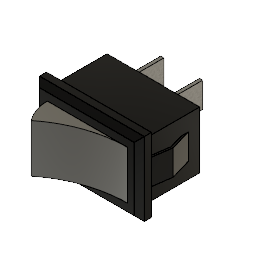
Irrigation unit - Rectangular On-off switch v1 (Autodesk Fusion 360 design; units mm, degrees)
Autodesk Fusion 360 part; units mm, degrees
note: some values were not read from the file. Set by a fixed rule: which face or edge a step refers to.
sketch "Sketch1" plane through (0, 0, 0) normal (0, 1, 0) x (1, 0, 0)
  line L0 (-0.7248, -15.1125) -> (17.4752, -15.1125)
  line L1 (17.4752, -15.1125) -> (17.4752, -3.8625)
  line L2 (17.4752, -3.8625) -> (-0.7248, -3.8625)
  line L3 (-0.7248, -3.8625) -> (-0.7248, -15.1125)
  line L4 (-1.9398, -16.7375) -> (18.6902, -16.7375)
  line L5 (18.6902, -16.7375) -> (18.6902, -2.2375)
  line L6 (18.6902, -2.2375) -> (-1.9398, -2.2375)
  line L7 (-1.9398, -2.2375) -> (-1.9398, -16.7375)
  line L8 (18.6902, -9.4875) -> (-20.1398, -9.4875) construction
  line L9 (8.3752, -16.7375) -> (8.3752, -13.4875) construction
  dimension "d727" = 18.2
  dimension "d728" = 11.25
  dimension "d729" = 14.5
  dimension "d730" = 20.63
  measures "d727" distance of L1 L3
  measures "d728" distance of L0 L2
  measures "d729" distance of L4 L6
  measures "d730" distance of L5 L7
extrude "Extrude1" add sketch "Sketch1" along normal blind 10.7 contours L0 L1 L2 L3 makes body 1
extrude "Extrude2" add sketch "Sketch1" against normal blind 2.4 contours L0 L1 L2 L3 | L4 L5 L6 L7 bodies 1
chamfer "Chamfer1" distance 1 angle 45 4 edges at (8.3752, -2.4, 16.7375) (-1.9398, -2.4, 9.4875) (8.3752, -2.4, 2.2375) (18.6902, -2.4, 9.4875) on bodies 1
sketch "Sketch2" plane through (17.4752, 0, 0) normal (1, 0, 0) x (0, 0, -1)
  line L0 (-15.1125, 0) -> (-3.8625, 0)
  line L1 (-3.8625, 0) -> (-3.8625, 10.7)
  line L2 (-3.8625, 10.7) -> (-15.1125, 10.7)
  line L3 (-15.1125, 10.7) -> (-15.1125, 0)
  line L4 (-11.9875, 0) -> (-6.9875, 0)
  line L5 (-6.9875, 0) -> (-6.9875, 8.5)
  line L6 (-6.9875, 8.5) -> (-11.9875, 8.5)
  line L7 (-11.9875, 8.5) -> (-11.9875, 0)
  line L8 (-16.7375, 0) -> (-2.2375, 0)
  dimension "d736" = 8.5
  dimension "d737" = 5
  measures "d736" distance of L6 L8
  measures "d737" distance of L5 L7
extrude "Extrude3" add sketch "Sketch2" along normal up to surface (1.215 mm away) separate body contours L0 L4 L5 L6 L7 L8 makes body 2
sketch "Sketch3" plane through (0, 0, 11.9875) normal (0, 0, 1) x (1, 0, 0)
  line L0 (18.6902, 0) -> (18.6902, 8.5)
  line L1 (18.6902, 8.5) -> (17.4752, 8.5)
  line L2 (18.6902, 4.25) -> (17.4752, 8.5)
  line L3 (18.6902, 4.25) -> (18.0827, 0)
  line L4 (17.4752, 7.0861) -> (18.2811, 4.2671)
  line L5 (18.2811, 4.2671) -> (17.5547, -0.8149)
  line L6 (17.4752, 8.5) -> (17.4752, 0)
  line L7 (17.4752, 0) -> (18.6902, 0)
extrude "Extrude5" cut sketch "Sketch3" against normal up to surface (5 mm away) contours L0 L3 L7 | L0 L1 L2 | L4 L5 L6 L7 bodies 2
copy_body "CopyPasteBodies1" bodies 2 makes body 3
move_body "Move1" bodies 3 to x (-1, 0, 0) y (0, 1, 0) z (0, 0, -1) at (34.9503, 0, 13.9751)
move_body "Move2" bodies 3 to x (1, 0, 0) y (0, 1, 0) z (0, 0, 1) at (-18.004, 0, 5)
combine "Combine1" operation add target body 1 tool bodies 2 3
sketch "Sketch4" plane through (0, 10.7, 0) normal (0, 1, 0) x (-1, 0, 0)
  line L0 (0.7248, 3.8625) -> (0.7248, 15.1125)
  line L1 (0.7248, 15.1125) -> (-17.4752, 15.1125)
  line L2 (-17.4752, 15.1125) -> (-17.4752, 3.8625)
  line L3 (-17.4752, 3.8625) -> (0.7248, 3.8625)
  line L4 (-1.8252, 11.9875) -> (-2.4752, 11.9875)
  line L5 (-2.4752, 11.9875) -> (-2.4752, 6.9875)
  line L6 (-2.4752, 6.9875) -> (-1.8252, 6.9875)
  line L7 (-1.8252, 6.9875) -> (-1.8252, 11.9875)
  line L8 (0.7248, 3.8625) -> (0.7248, 15.1125)
  line L9 (-18.6902, 9.4875) -> (20.1398, 9.4875)
  dimension "d744" = 0.65
  dimension "d745" = 5
  dimension "d746" = 3.2
  measures "d744" distance of L5 L7
  measures "d745" distance of L4 L6
  measures "d746" distance of L5 L8
extrude "Extrude6" add sketch "Sketch4" along normal blind 8 separate body contours L4 L5 L7 L9 | L5 L6 L7 L9 makes body 4
copy_body "CopyPasteBodies2" bodies 4 makes body 5
move_body "Move3" bodies 5 to x (1, 0, 0) y (0, 1, 0) z (0, 0, 1) at (7.6, 0, 0)
sketch "Sketch5" plane through (0, -2.4, 0) normal (0, -1, 0) x (1, 0, 0)
  line L0 (-0.9398, 3.2375) -> (17.6902, 3.2375)
  line L1 (17.6902, 3.2375) -> (17.6902, 15.7375)
  line L2 (17.6902, 15.7375) -> (-0.9398, 15.7375)
  line L3 (-0.9398, 15.7375) -> (-0.9398, 3.2375)
  line L4 (0.3752, 4.7375) -> (16.3752, 4.7375)
  line L5 (16.3752, 4.7375) -> (16.3752, 14.2375)
  line L6 (16.3752, 14.2375) -> (0.3752, 14.2375)
  line L7 (0.3752, 14.2375) -> (0.3752, 4.7375)
  line L8 (18.6902, 9.4875) -> (-20.1398, 9.4875)
  line L9 (8.3752, 16.7375) -> (8.3752, 13.4875)
  dimension "d749" = 9.5
  dimension "d750" = 16
  measures "d749" distance of L4 L6
  measures "d750" distance of L5 L7
extrude "Extrude7" add sketch "Sketch5" along normal blind 4.9 separate body contours L4 L5 L7 L8 | L5 L6 L7 L8 makes body 6
sketch "Sketch6" plane through (0, 0, 4.7375) normal (0, 0, -1) x (-1, 0, 0)
  line L0 (-0.3752, -2.4) -> (-16.3752, -2.4)
  line L1 (-16.3752, -2.4) -> (-16.3752, -7.3)
  line L2 (-16.3752, -7.3) -> (-0.3752, -7.3)
  line L3 (-0.3752, -7.3) -> (-0.3752, -2.4)
  arc A0 (-2.3366, -7.3) -> (-16.3752, -2.4) centre (-8.5008, -2.4) ccw
  arc A1 (-2.3366, -7.3) -> (-16.3752, -2.4) centre (-16.3752, -24.9602) ccw
extrude "Extrude8" cut sketch "Sketch6" against normal up to surface (9.5 mm away) contours L0 L2 L3 A0 | L1 L2 A1 bodies 6
